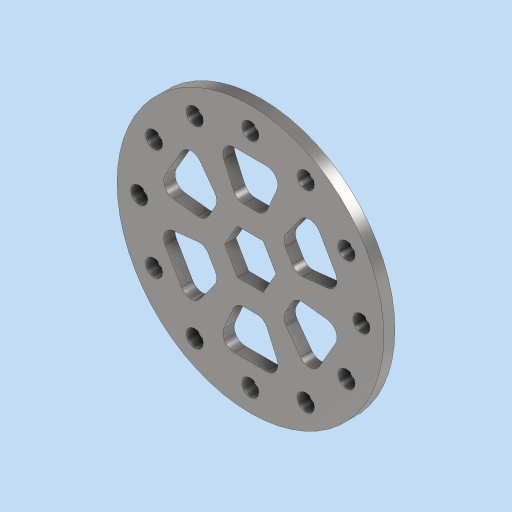
# Autodesk Inventor part: ThickWheelPlate_v83DPrintable
Saved by Autodesk Inventor 2023 (Build 270158000, 158)
## iProperties
Created: 2023-04-06
Part Number: ThickWheelPlate_v83DPrintable
Material: Steel, Alloy
Document SubType Name: Modeling
Designer: asach
Density: 7.73 g/cm^3
Appearance: Semi-Polished
Author: asach
Autodesk Inventor part; units mm, degrees
ref_plane "YZ Plane" through (0, 0, 0) normal (1, 0, 0) x (0, 1, 0)
ref_plane "XZ Plane" through (0, 0, 0) normal (0, 1, 0) x (-1, 0, 0)
ref_plane "XY Plane" through (0, 0, 0) normal (0, 0, 1) x (1, 0, 0)
sketch "Sketch1" plane through (0, 0, 0) normal (0, 0, 1) x (1, 0, 0)
  circle A0 centre (0, 0) radius 38.1
  line L0 (7.3323, 0) -> (3.6662, -6.35)
  line L1 (3.6662, -6.35) -> (-3.6662, -6.35)
  line L2 (-3.6662, -6.35) -> (-7.3323, 0)
  line L3 (-7.3323, 0) -> (-3.6662, 6.35)
  line L4 (-3.6662, 6.35) -> (3.6662, 6.35)
  line L5 (3.6662, 6.35) -> (7.3323, 0)
  circle A1 centre (0, 0) radius 31.75 construction
  circle A2 centre (0, 31.75) radius 2.413
  circle A3 centre (-15.875, 27.4963) radius 2.413
  circle A4 centre (-27.4963, 15.875) radius 2.413
  circle A5 centre (-31.75, 0) radius 2.413
  circle A6 centre (-27.4963, -15.875) radius 2.413
  circle A7 centre (-15.875, -27.4963) radius 2.413
  circle A8 centre (0, -31.75) radius 2.413
  circle A9 centre (15.875, -27.4963) radius 2.413
  circle A10 centre (27.4963, -15.875) radius 2.413
  circle A11 centre (31.75, 0) radius 2.413
  circle A12 centre (27.4963, 15.875) radius 2.413
  circle A13 centre (15.875, 27.4963) radius 2.413
  line L6 (-9.525, 25.4) -> (-3.9688, 12.7)
  line L7 (-3.9688, 12.7) -> (3.9688, 12.7)
  line L8 (3.9688, 12.7) -> (9.525, 25.4)
  line L9 (9.525, 25.4) -> (-9.525, 25.4)
  line L10 (0, -53.34) -> (0, 53.34) construction
  circle A14 centre (0, 0) radius 25.4 construction
  line L11 (0, 29.337) -> (0, 25.4)
  line L12 (0, 38.1) -> (0, 25.4)
  dimension "d0" = 76.2
  dimension "d2" = 63.5
  dimension "d3" = 4.826
  dimension "d1" = 12.7
  dimension "d6" = 360
  dimension "d16" = 6.35
  dimension "d18" = 7.9375
  dimension "d19" = 19.05
  dimension "d20" = 12.7
  constraints: 24 end point, 11 centre point, 4 coincident, 4 vertical alignment, 2 point on line, 1 collinear, 1 equal length, 1 horizontal, 1 midpoint, 1 parallel, 1 perpendicular, 46 other
  measures "d1" distance between parallel lines of L1 L4
  measures "d16" distance between parallel lines of L4 L7
  measures "d18" distance of L6.end L7.end
  measures "d19" distance of L8.end L6.start
  measures "d20" distance of L12.start L11.end
extrude "Extrusion1" add sketch "Sketch1" along normal blind 3.175 contours A0 | L9 L8 L7 L6
extrude "Extrusion2" cut sketch "Sketch1" along normal blind 3.175 contours L9 L8 L7 L6
fillet "Fillet1" radius 3.175 4 edges at (-9.525, 25.4, 1.5875) (9.525, 25.4, 1.5875) (-3.9688, 12.7, 1.5875) (3.9688, 12.7, 1.5875)
pattern_circular "Circular Pattern1" count 6 over 360 about axis through (0, 0, 0) along (0, 0, 1) of "Extrusion2", "Fillet1"
body "Solid1"
